Autodesk Inventor part; units mm, degrees
(part 2 of 2)
  line L121 (6.1961, 43.2003) -> (8.3839, 43.2003)
  point P0 (0, 0)
  constraints: 2 other
extrude "Extrusion16" cut sketch "Sketch15" against normal blind 4
sketch "Sketch16" plane through (-93.3464, 30, 62.7) normal (0, 0, 1) x (1, 0, 0)
  line L0 (6.6464, 0) -> (6.6464, -15) projected
  line L1 (160.0464, -15) -> (160.0464, 0) projected
  line L2 (166.6929, 0) -> (166.6929, -23) projected
  line L3 (0, 0) -> (166.6929, 0) projected
  line L4 (0, -23) -> (0, 0) projected
  line L5 (166.6929, -23) -> (0, -23) projected
  line L6 (160.0464, 0) -> (6.6464, 0) projected
  line L7 (6.6464, -15) -> (160.0464, -15) projected
  line L8 (6.6464, -7.5) -> (45.8464, -7.5) construction
  arc A0 (40.8464, -7.5) -> (50.8464, -7.5) centre (45.8464, -7.5) ccw
  line L9 (45.8464, -7.5) -> (70.8464, -7.5) construction
  line L10 (70.8464, -7.5) -> (95.8464, -7.5) construction
  line L11 (95.8464, -7.5) -> (120.8464, -7.5) construction
  arc A1 (65.8464, -7.5) -> (75.8464, -7.5) centre (70.8464, -7.5) ccw
  arc A2 (90.8464, -7.5) -> (100.8464, -7.5) centre (95.8464, -7.5) ccw
  arc A3 (115.8464, -7.5) -> (125.8464, -7.5) centre (120.8464, -7.5) ccw
  line L12 (40.8464, -7.5) -> (40.8464, 0)
  line L13 (40.8464, 0) -> (50.8464, 0)
  line L14 (50.8464, -7.5) -> (50.8464, 0)
  line L15 (65.8464, -7.5) -> (65.8464, 0)
  line L16 (65.8464, 0) -> (75.8464, 0)
  line L17 (75.8464, -7.5) -> (75.8464, 0)
  line L18 (90.8464, -7.5) -> (90.8464, 0)
  line L19 (90.8464, 0) -> (100.8464, 0)
  line L20 (100.8464, -7.5) -> (100.8464, 0)
  line L21 (115.8464, -7.5) -> (115.8464, 0)
  line L22 (115.8464, 0) -> (125.8464, 0)
  line L23 (125.8464, -7.5) -> (125.8464, 0)
  point P0 (93.3464, -30)
  dimension "d241" = 153.4
  dimension "d242" = 39.2
  dimension "d243" = 10
  dimension "d244" = 25
  dimension "d245" = 25
  dimension "d246" = 25
  dimension "d247" = 10
  dimension "d248" = 10
  dimension "d249" = 10
  constraints: 32 end point, 8 point on circle, 8 point on line, 8 tangent, 7 perpendicular, 4 centre point, 4 coincident, 2 horizontal, 1 midpoint, 1 vertical, 9 other
  measures "d241" distance between parallel lines of L1 L0
  measures "d242" distance of L8.start L8.end
  measures "d243" diameter of A0
  measures "d244" distance of L9.start L9.end
  measures "d245" distance of L9.end L10.end
  measures "d246" distance of L10.end L11.end
  measures "d247" diameter of A1
  measures "d248" diameter of A2
  measures "d249" diameter of A3
extrude "Extrusion17" cut sketch "Sketch16" against normal through all contours L3 L14 A0 L12 | L3 L17 A1 L15 | L23 A3 L21 L3 | L3 L20 A2 L18
body "Solid1"
